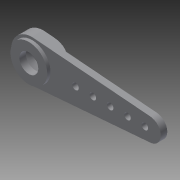
# Autodesk Inventor part: servo_arm_2
Saved by Autodesk Inventor 2015 SP2 (Build 190223200, 223)
## iProperties
Created: 2016-09-05
Part Number: servo_arm_2
Material: Generic
Document SubType Name: Modeling
Designer: jm799
Density: 1 g/cm^3
Appearance: Default
Author: jm799
Autodesk Inventor part; units mm, degrees
ref_plane "YZ Plane" through (0, 0, 0) normal (1, 0, 0) x (0, 1, 0)
ref_plane "XZ Plane" through (0, 0, 0) normal (0, 1, 0) x (-1, 0, 0)
ref_plane "XY Plane" through (0, 0, 0) normal (0, 0, 1) x (1, 0, 0)
sketch "Sketch1" plane through (0, 0, 0) normal (0, 1, 0) x (-1, 0, 0)
  circle A0 centre (0, 0) radius 6.45
  circle A1 centre (0, 0) radius 5.657
  circle A2 centre (0, 0) radius 2.85
  circle A3 centre (0, 0) radius 1.5
  line L0 (0, 0) -> (-36, 0)
  circle A4 centre (-36, 0) radius 3.5
  line L1 (0, 6.45) -> (-36, 3.5)
  line L2 (0, -6.45) -> (-36, -3.5)
  dimension "d0" = 12.9
  dimension "d1" = 11.314
  dimension "d2" = 5.7
  dimension "d3" = 3
  dimension "d4" = 36
  dimension "d5" = 7
  constraints: 6 end point, 5 centre point, 5 coincident, 4 point on circle, 1 horizontal
  measures "d0" diameter of A0
  measures "d1" diameter of A1
  measures "d2" diameter of A2
  measures "d3" diameter of A3
  measures "d4" distance of L0.start L0.end
  measures "d5" diameter of A4
extrude "Extrusion1" add sketch "Sketch1" along normal blind 2 contours A0 L2 L1 | A0 L0 A4 L1 | L2 A4 L0 A0 | A4
sketch "Sketch2" plane through (0, 2, 0) normal (0, 1, 0) x (1, 0, 0)
  line L0 (8.4358, -5.7587) -> (8.4358, 5.7587)
  line L1 (8.4358, -5.7587) -> (0, -6.45)
  line L2 (0, -6.45) -> (36, -3.5) projected
  line L3 (8.4358, 5.7587) -> (0, 6.45)
  line L4 (36, 3.5) -> (0, 6.45) projected
  arc A0 (0, 6.45) -> (0, -6.45) centre (0, 0) ccw
  arc A1 (0, 6.45) -> (0, -6.45) centre (0, 0) ccw projected
  circle A2 centre (0, 0) radius 5.657
  constraints: 6 end point, 2 centre point, 2 collinear, 2 point on circle, 1 coincident, 1 concentric, 1 vertical
extrude "Extrusion2" add sketch "Sketch2" along normal blind 1.5
fillet "Fillet1" radius 10 1 edges at (8.4358, 3.5, 0)
sketch "Sketch4" plane through (0, 2, 0) normal (0, 1, 0) x (1, 0, 0)
  circle A0 centre (0, 0) radius 2.9
  circle A1 centre (0, 0) radius 1.5
  dimension "d11" = 5.8
  dimension "d12" = 3
  constraints: 2 centre point, 2 coincident
  measures "d11" diameter of A0
  measures "d12" diameter of A1
sketch "Sketch5" plane through (0, 2, 0) normal (0, 1, 0) x (1, 0, 0)
  circle A0 centre (0, 0) radius 5.657
  constraints: 1 centre point
extrude "Extrusion3" add sketch "Sketch5" along normal blind 0.5 and the other way blind 3
sketch "Sketch6" plane through (0, 2.5, 0) normal (0, 1, 0) x (1, 0, 0)
  circle A0 centre (0, 0) radius 2.9
  dimension "d17" = 5.8
  constraints: 1 centre point, 1 coincident
  measures "d17" diameter of A0
extrude "Extrusion4" cut sketch "Sketch6" against normal blind 0.5
hole "Hole1" at (0, 2, 0) direction (0, -1, 0) diameter 3 end through all
sketch "Sketch7" plane through (0, -1, 0) normal (0, -1, 0) x (1, 0, 0)
  circle A0 centre (0, 0) radius 2.9
  dimension "d27" = 5.8
  constraints: 1 centre point, 1 coincident
  measures "d27" diameter of A0
hole "Hole2" at (0, -1, 0) direction (0, 1, 0) diameter 5.8 depth 2 tip angle 118
sketch "Sketch9" plane through (0, 2, 0) normal (0, 1, 0) x (1, 0, 0)
  line L0 (8.4358, 5.7587) -> (8.4358, -5.7587) projected
  arc A0 (36, -3.5) -> (36, 3.5) centre (36, 0) ccw projected
  circle A1 centre (23.9679, 0) radius 1
  circle A2 centre (34.612, 0) radius 1
  line L1 (0, -6.45) -> (36, -3.5) projected
  circle A3 centre (29.29, 0) radius 1
  circle A4 centre (13.3238, 0) radius 1
  circle A5 centre (18.6459, 0) radius 1
  point P0 (0, 0)
  constraints: 5 centre point
hole "Hole4" at (13.3238, 2, 0) at (18.6459, 2, 0) at (23.9679, 2, 0) at (29.29, 2, 0) at (34.612, 2, 0) direction (0, -1, 0) diameter 2 end through all
body "Solid1"
